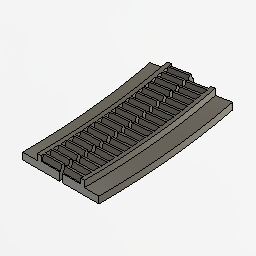
Rack2_Curved (Autodesk Fusion 360 design; units mm, degrees)
Autodesk Fusion 360 part; units mm, degrees
sketch "Curve Base Shape" plane through (0, 0, 0) normal (0, 0, 1) x (1, 0, 0) in component "Rack2 Curved"
  arc A0 (0, 0) -> (-6.1487, 62.4289) centre (-320, 0) ccw construction
  line L0 (-8, 0) -> (8, 0) construction
  line L1 (-13.995, 60.8682) -> (1.6976, 63.9896) construction
  arc A1 (-8, 0) -> (-13.995, 60.8682) centre (-320, 0) ccw construction
  arc A2 (8, 0) -> (1.6976, 63.9896) centre (-320, 0) ccw construction
  line L2 (-9.5024, 30.5813) -> (6.4206, 32.1496) construction
  dimension "d104" = 11.25
  dimension "d109" = 8
  dimension "d110" = 8
  dimension "d111" = 320
  measures "d104" angle of L0 L1
  measures "d109" distance of A0 A2
  measures "d110" distance of A0 A1
  measures "d111" radius of A0
sketch "Curve Base" plane through (0, 0, 0) normal (0, 0, 1) x (1, 0, 0) in component "Rack2 Curved"
  arc A0 (-8, 0) -> (-13.995, 60.8682) centre (-320, 0) ccw construction
  line L0 (-8, 0) -> (8, 0) construction
  arc A1 (8, 0) -> (1.6976, 63.9896) centre (-320, 0) ccw construction
  line L1 (-13.995, 60.8682) -> (1.6976, 63.9896) construction
  line L2 (-9.5024, 30.5813) -> (6.4206, 32.1496) construction
  arc A2 (7.9, 0.1) -> (1.619, 63.872) centre (-320, 0) ccw
  arc A3 (-7.9, 0.1) -> (-13.8774, 60.7896) centre (-320, 0) ccw
  line L3 (-13.8774, 60.7896) -> (1.619, 63.872)
  line L4 (-7.9, 0.1) -> (7.9, 0.1)
  circle A4 centre (4, 4) radius 2.475 construction
  line L5 (-6.475, 1.525) -> (6.475, 1.525)
  line L6 (6.475, 1.525) -> (6.475, 6.475)
  line L7 (6.475, 6.475) -> (-6.475, 6.475)
  line L8 (-6.475, 6.475) -> (-6.475, 1.525)
  line L9 (0, 1.525) -> (0, 6.475) construction
  line L10 (-11.2361, 54.8151) -> (-12.2018, 59.67)
  line L11 (-12.2018, 59.67) -> (0.4994, 62.1964)
  line L12 (1.4651, 57.3415) -> (-11.2361, 54.8151)
  line L13 (0.4994, 62.1964) -> (1.4651, 57.3415)
  circle A5 centre (2.0478, 35.7383) radius 2.475 construction
  line L14 (-2.1755, 37.8093) -> (-1.5409, 31.3655) construction
  line L15 (-8.6194, 37.1746) -> (4.2683, 38.444)
  line L16 (4.2683, 38.444) -> (5.5376, 25.5563)
  line L17 (5.5376, 25.5563) -> (-7.35, 24.287)
  line L18 (-7.35, 24.287) -> (-8.6194, 37.1746)
  circle A6 centre (-1.5409, 31.3655) radius 3.1819
  circle A7 centre (-1.5409, 31.3655) radius 1.7819
  dimension "d112" = 0.1
  dimension "d114" = 0.1
  dimension "d115" = 0.1
  dimension "d116" = 0.1
  dimension "d117" = 4
  dimension "d118" = 4.95
  dimension "d119" = 4
  dimension "d120" = 4.95
  dimension "d121" = 4
  dimension "d122" = 4
  dimension "d123" = 1.4
  measures "d112" distance of L1 L3
  measures "d114" distance of A1 A2
  measures "d115" distance of A0 A3
  measures "d116" distance of L0 L4
  measures "d117" distance of L0 A4.centre
  measures "d118" diameter of A4
  measures "d119" distance of origin A4.centre
  measures "d120" diameter of A5
  measures "d121" distance of L2 A5.centre
  measures "d122" distance of A5.centre L14
  measures "d123" distance of A6 A7
sketch "Section" plane through (0, 0, 0) normal (0, 1, 0) x (1, 0, 0) in component "Rack2 Curved"
  line L0 (-8, -5.9) -> (8, -5.9)
  line L1 (8, -5.9) -> (8, 0)
  line L2 (-8, 0) -> (-8, -5.9)
  line L3 (0, 0) -> (0, -5.9) construction
  line L4 (-320, -5.9) -> (-320, 0) construction
  line L5 (1.6, -5.9) -> (1.6, -3.2)
  line L6 (1.6, -3.2) -> (8, -3.2)
  line L7 (-1.6, -5.9) -> (-1.6, -3.2)
  line L8 (-1.6, -3.2) -> (-8, -3.2)
  line L9 (0, -2.3) -> (6.475, -2.3) construction
  line L10 (6.475, -2.3) -> (6.475, 0) construction
  line L11 (-6.475, 0) -> (-6.475, -1.8) construction
  line L12 (-6.475, -1.8) -> (-1.525, -1.8) construction
  line L13 (-1.525, -1.8) -> (-1.525, 0) construction
  line L14 (-8, 0) -> (8, 0)
  point P0 (-4, -1.8)
  dimension "d74" = 5.9
  dimension "d76" = 320
  dimension "d78" = 1.6
  dimension "d98" = 4.95
  dimension "d99" = 4
  dimension "d100" = 1.8
  dimension "d101" = 0.9
  dimension "d102" = 0.5
  dimension "d124" = 3.2
  measures "d74" distance of L0.end L1.end
  measures "d76" distance of L3.start L4.end
  measures "d78" distance of L3 L5
  measures "d98" distance of L11.end L12.end
  measures "d99" distance of L3 P0
  measures "d100" distance of L11.start L11.end
  measures "d101" distance of L6 L9
  measures "d102" distance of L9 L12
  measures "d124" distance of L6.end L14
sketch "Tooth A" plane through (0, 0, 0) normal (1, 0, 0) x (0, 1, 0) in component "Rack2 Curved"
  line L0 (0, 0) -> (0, 5.9) construction
  line L1 (0, 5.9) -> (1.2986, 5.9)
  line L2 (1.2986, 5.9) -> (0.5342, 3.8)
  line L3 (0.5342, 3.8) -> (0, 3.8)
  line L4 (0, 4.85) -> (0.9164, 4.85) construction
  line L5 (0, 5.9) -> (-1.2986, 5.9)
  line L6 (-1.2986, 5.9) -> (-0.5342, 3.8)
  line L7 (-0.5342, 3.8) -> (0, 3.8)
  dimension "d87" = 3.8
  dimension "d88" = 20
  dimension "d89" = 0.9164
  measures "d87" distance of L0.start L3
  measures "d88" angle of L0 L2
  measures "d89" distance of L4.start L4.end
sketch "Tooth B" plane through (0, 0, 0) normal (1, 0, 0) x (0, 1, 0) in component "Rack2 Curved"
  line L0 (0, 0) -> (0, 5.9) construction
  line L1 (0, 5.9) -> (1.2774, 5.9)
  line L2 (1.2774, 5.9) -> (0.513, 3.8)
  line L3 (0.513, 3.8) -> (0, 3.8)
  line L4 (0.8952, 4.85) -> (0, 4.85) construction
  line L5 (0, 5.9) -> (-1.2774, 5.9)
  line L6 (-1.2774, 5.9) -> (-0.513, 3.8)
  line L7 (-0.513, 3.8) -> (0, 3.8)
  dimension "d138" = 20
  dimension "d139" = 0.8952
  dimension "d140" = 3.8
  measures "d138" angle of L0 L2
  measures "d139" distance of L4.start L4.end
  measures "d140" distance of L0.start L3
extrude "Extrude2" add sketch "Curve Base" along normal up to surface (5.9 mm away) contours A2 A3 L3 L4 | L5 L6 L7 L8 | L10 L11 L12 L13 | L15 L16 L17 L18 | A6 | A7 makes body 1 in component "Rack2 Curved"
revolve "Revolve2" cut sketch "Section" angle 360 about axis through (-320, 0, 5.9) along (0, 0, -1) contours L0 L1 L5 L6 bodies 1 in component "Rack2 Curved"
extrude "Extrude4" cut sketch "Curve Base" along normal up to surface (2.3 mm away) contours L5 L6 L7 L8 | L10 L11 L12 L13 bodies 1 in component "Rack2 Curved"
chamfer "Chamfer2" distance 0.3 angle 45 12 edges at (-5.8512, 60.9332, 0) (-11.7189, 57.2426, 0) (-4.8855, 56.0783, 0) (0.9822, 59.769, 0) (-9.4028, 30.5911, 0) (-6.1292, 62.3308, 0) (6.3211, 32.1398, 0) (0, 0.1, 0) (0, 1.525, 0) (-6.475, 4, 0) (0, 6.475, 0) (6.475, 4, 0) on bodies 1 in component "Rack2 Curved"
extrude "Extrude5" cut sketch "Curve Base" along normal up to surface (2.3 mm away) contours L15 L16 L17 L18 | A7 bodies 1 in component "Rack2 Curved"
chamfer "Chamfer1" distance 0.3 angle 45 6 edges at (-7.9847, 30.7308, 0) (-2.1755, 37.8093, 0) (4.9029, 32.0001, 0) (-0.9062, 24.9217, 0) (-3.2022, 30.7211, 0) (-4.5074, 32.5161, 0) on bodies 1 in component "Rack2 Curved"
pattern_circular "C-Pattern2" count 3 over 5.625 about axis through (-320, 0, 0) along (0, 0, 1) both ways of "Extrude5", "Chamfer1" in component "Rack2 Curved"
extrude "Extrude3" cut sketch "Tooth A" against normal up to surface (8 mm away) bodies 1 in component "Rack2 Curved"
pattern_circular "C-Pattern1" count 19 over 11.25 about axis through (-320, 0, 0.3) along (0, 0, 1) of "Extrude3" in component "Rack2 Curved"
extrude "Extrude6" add sketch "Curve Base" along normal up to surface (5.9 mm away) separate body contours A2 A3 L3 L4 | L5 L6 L7 L8 | L10 L11 L12 L13 | L15 L16 L17 L18 | A6 | A7 makes body 2 in component "Rack2 Curved"
revolve "Revolve3" cut sketch "Section" angle 360 about axis through (-320, 0, 5.9) along (0, 0, -1) contours L0 L2 L7 L8 bodies 2 in component "Rack2 Curved"
extrude "Extrude7" cut sketch "Curve Base" along normal up to surface (2.3 mm away) contours L5 L6 L7 L8 | L10 L11 L12 L13 bodies 2 in component "Rack2 Curved"
chamfer "Chamfer3" distance 0.3 angle 45 12 edges at (-4.8855, 56.0783, 0) (0.9822, 59.769, 0) (-5.8512, 60.9332, 0) (6.3211, 32.1398, 0) (-6.1292, 62.3308, 0) (-11.7189, 57.2426, 0) (-9.4028, 30.5911, 0) (0, 0.1, 0) (0, 1.525, 0) (6.475, 4, 0) (0, 6.475, 0) (-6.475, 4, 0) on bodies 2 in component "Rack2 Curved"
extrude "Extrude8" cut sketch "Curve Base" along normal up to surface (2.3 mm away) contours L15 L16 L17 L18 | A7 bodies 2 in component "Rack2 Curved"
chamfer "Chamfer4" distance 0.3 angle 45 6 edges at (-4.5074, 32.5161, 0) (-3.2022, 30.7211, 0) (4.9029, 32.0001, 0) (-0.9062, 24.9217, 0) (-2.1755, 37.8093, 0) (-7.9847, 30.7308, 0) on bodies 2 in component "Rack2 Curved"
pattern_circular "C-Pattern3" count 3 over 5.625 about axis through (-320, 0, 0) along (0, 0, 1) both ways of "Extrude8", "Chamfer4" in component "Rack2 Curved"
extrude "Extrude9" cut sketch "Tooth B" along normal up to surface (8 mm away) bodies 2 in component "Rack2 Curved"
pattern_circular "C-Pattern4" count 20 over 11.25 about axis through (-320, 0, 5.9) along (0, 0, 1) of "Extrude9" in component "Rack2 Curved"
move_body "Move1" bodies 2 to x (1, 0, 0) y (0, 1, 0) z (0, 0, 1) at (-17, 0, 0) in component "Rack2 Curved"
component "Rack2 Curved" placed x (1, 0, 0) y (0, 1, 0) z (0, 0, 1) at (0, 0, 0)
equation "DeltaX = 8 mm"
equation "DeltaY = 8 mm"
equation "DeltaZ = 3.2 mm"
equation "Wall = 0.8 mm"
equation "Gap = 0.1 mm"
equation "KnobDiameter = 4.95 mm"
equation "KnobHeight = 1.8 mm"
equation "WallZ = 1 mm"
equation "BasePlateChamfer = 0.3 mm"
equation "CurveRadius = 40"
equation "CurveAngle = ( 90 / 8 ) * 1 deg"
equation "Height = 5.9 mm"
equation "BaseHeight = 3.8 mm"
equation "d74 = Height"
equation "d76 = CurveRadius * DeltaX"
equation "Module = 1 mm"
equation "CurveLengthA = ( PI * CurveAngle / 180 deg ) * DeltaX * ( CurveRadius - 0.5 )"
equation "CurveLengthB = ( PI * CurveAngle / 180 deg ) * DeltaX * ( CurveRadius + 0.5 )"
equation "NumTeethA = floor(CurveLengthA / ( PI * Module ))"
equation "NumTeethB = floor(CurveLengthB / ( PI * Module ))"
equation "PressureAngle = 20 deg"
equation "d87 = BaseHeight"
equation "d88 = PressureAngle"
equation "d89 = CurveLengthA / NumTeethA / 4 + Gap"
equation "d92 = NumTeethA"
equation "d93 = CurveAngle"
equation "d98 = KnobDiameter"
equation "d99 = DeltaX / 2"
equation "d100 = KnobHeight"
equation "d101 = ( 6 * 0.15 ) * 1 mm"
equation "d104 = CurveAngle"
equation "d109 = DeltaX"
equation "d110 = DeltaX"
equation "d111 = CurveRadius * DeltaX"
equation "d112 = Gap"
equation "d114 = Gap"
equation "d115 = Gap"
equation "d116 = Gap"
equation "d117 = DeltaY / 2"
equation "d118 = KnobDiameter"
equation "d119 = DeltaX / 2"
equation "d120 = KnobDiameter"
equation "d121 = DeltaY / 2"
equation "d122 = DeltaX / 2"
equation "d123 = 0.8 mm + 2 * BasePlateChamfer"
equation "d124 = DeltaZ"
equation "d135 = CurveAngle / 2"
equation "d136 = BasePlateChamfer"
equation "d137 = BasePlateChamfer"
equation "d138 = PressureAngle"
equation "d139 = CurveLengthB / NumTeethB / 4 + Gap"
equation "d140 = BaseHeight"
equation "d146 = BasePlateChamfer"
equation "d149 = BasePlateChamfer"
equation "d151 = CurveAngle / 2"
equation "d154 = NumTeethB"
equation "d155 = -CurveAngle"
named bodies: "Rack2 Curved B", "Rack2 Curved C"
